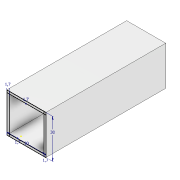
# Autodesk Inventor part: Cablecanal Ranurado 30x30 L=116 mm
Saved by Autodesk Inventor 2020 (Build 240168000, 168)
## iProperties
Created: 2020-07-11
Part Number: Cablecanal Ranurado 30x30 L=116 mm
Material: PPS Plastic
Document SubType Name: Modeling
Designer: Hernan
Density: 1.637 g/cm^3
Appearance: Smooth - White
Author: Hernan
Autodesk Inventor part; units mm, degrees
ref_plane "YZ Plane" through (0, 0, 0) normal (1, 0, 0) x (0, 1, 0)
ref_plane "XZ Plane" through (0, 0, 0) normal (0, 1, 0) x (-1, 0, 0)
ref_plane "XY Plane" through (0, 0, 0) normal (0, 0, 1) x (1, 0, 0)
sketch "Sketch1" plane through (0, 0, 0) normal (0, 0, 1) x (1, 0, 0)
  line L0 (-10.947, -4.6264) -> (19.053, -4.6264)
  line L1 (19.053, -4.6264) -> (19.053, 25.3736)
  line L2 (19.053, 25.3736) -> (-10.947, 25.3736)
  line L3 (-10.947, 25.3736) -> (-10.947, -4.6264)
  line L4 (-10.947, 23.6736) -> (19.053, 23.6736)
  line L5 (-9.247, -4.6264) -> (-9.247, 25.3736)
  line L6 (17.353, -4.6264) -> (17.353, 25.3736)
  line L7 (-10.947, -2.9264) -> (19.053, -2.9264)
  point P0 (0, 0)
  point P1 (-9.247, -2.9264)
  point P2 (17.353, -2.9264)
  point P3 (17.353, 23.6736)
  point P4 (-9.247, 23.6736)
  dimension "d0" = 30
  dimension "d1" = 30
  dimension "d2" = 1.7
  dimension "d3" = 1.7
  dimension "d4" = 1.7
  dimension "d5" = 1.7
  constraints: 16 end point, 8 point on line, 3 horizontal, 2 perpendicular, 2 vertical, 1 parallel
  measures "d0" distance of L0.start L0.end
  measures "d1" distance of L0.end L1.end
  measures "d2" distance between parallel lines of L2 L4
  measures "d3" distance between parallel lines of L3 L5
  measures "d4" distance between parallel lines of L0 L7
  measures "d5" distance between parallel lines of L1 L6
extrude "Extrusion1" add sketch "Sketch1" against normal blind 92.042
extrude "Extrusion2" cut sketch "Sketch1" against normal blind 100000 contours L5 L4 L6 L7
body "Solid1"
